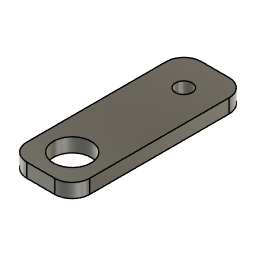
Shaft Connector (Autodesk Fusion 360 design; units mm, degrees)
Autodesk Fusion 360 part; units mm, degrees
sketch "Sketch1" plane through (0, 0, 0) normal (0, 0, 1) x (1, 0, 0)
  line L0 (-4.5, 12.5) -> (4.5, 12.5)
  line L1 (4.5, 12.5) -> (4.5, -12.5)
  line L2 (4.5, -12.5) -> (-4.5, -12.5)
  line L3 (-4.5, -12.5) -> (-4.5, 12.5)
  line L4 (-4.5, 12.5) -> (4.5, -12.5) construction
  line L5 (4.5, 12.5) -> (-4.5, -12.5) construction
  dimension "d1" = 9
  dimension "d2" = 25
  constraint horizontal L0
  constraint perpendicular L0 L1
  constraint parallel L0 L2
  constraint parallel L1 L3
  constraint coincident L4 origin
  constraint coincident L5 origin
  measures "d1" distance of L1.end L2.end
  measures "d2" distance of L0.end L1.end
extrude "Extrude1" add sketch "Sketch1" along normal blind 2
fillet "Fillet4" radius 2.5 4 edges at (4.5, 12.5, 1) (-4.5, 12.5, 1) (-4.5, -12.5, 1) (4.5, -12.5, 1)
sketch "Sketch7" plane through (0, 0, 2) normal (0, 0, 1) x (-1, 0, 0)
  arc A0 (-2, 12.5) -> (-4.5, 10) centre (-2, 10) ccw
  line L0 (-4.5, 10) -> (-4.5, -10)
  arc A1 (2, -12.5) -> (4.5, -10) centre (2, -10) ccw
  line L1 (4.5, -10) -> (4.5, 10)
  arc A2 (-4.5, -10) -> (-2, -12.5) centre (-2, -10) ccw
  line L2 (-2, -12.5) -> (2, -12.5)
  arc A3 (4.5, 10) -> (2, 12.5) centre (2, 10) ccw
  line L3 (2, 12.5) -> (-2, 12.5)
  line L4 (0, 12.5) -> (0, -12.5) construction
  line L5 (0, 12.5) -> (0, 8)
  line L6 (0, -12.5) -> (0, -8)
  circle A4 centre (0, -8) radius 1.2
  circle A5 centre (0, 8) radius 2.7
  dimension "d40" = 2.4
  dimension "d41" = 5.4
  constraint midpoint L3 L4.start
  constraint midpoint L2 L4.end
  constraint coincident L4 L5.end
  constraint perpendicular L3 L5
  constraint coincident L4 L6.end
  constraint coincident L6.end A4.centre
  constraint coincident L5.end A5.centre
  measures "d40" diameter of A4
  measures "d41" diameter of A5
extrude "Extrude7" cut sketch "Sketch7" against normal blind 3 contours A4 | A5
